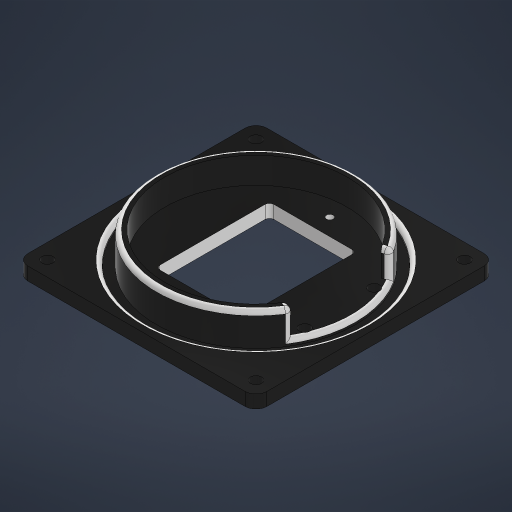
# Autodesk Inventor part: UnitV_Mount
Saved by Autodesk Inventor 2024.2 (Build 282272000, 272)
## iProperties
Created: 2024-02-19
Part Number: UnitV_Mount
Material: 一般
Document SubType Name: Modeling
Designer: Hanaoka
Density: 1 g/cm^3
Appearance: 既定
Author: Hanaoka
Autodesk Inventor part; units mm, degrees
ref_plane "YZ Plane" through (0, 0, 0) normal (1, 0, 0) x (0, 1, 0)
ref_plane "XZ Plane" through (0, 0, 0) normal (0, 1, 0) x (-1, 0, 0)
ref_plane "XY Plane" through (0, 0, 0) normal (0, 0, 1) x (1, 0, 0)
sketch "スケッチ1" plane through (0, 0, 0) normal (0, 1, 0) x (-1, 0, 0)
  line L0 (-24, 24) -> (24, 24) construction
  line L1 (24, 24) -> (24, -24) construction
  line L2 (24, -24) -> (-24, -24) construction
  line L3 (-24, -24) -> (-24, 24) construction
  line L4 (-24, 24) -> (24, -24) construction
  line L5 (24, 24) -> (-24, -24) construction
  line L6 (-25, 27.5) -> (25, 27.5)
  line L7 (27.5, 25) -> (27.5, -25)
  line L8 (25, -27.5) -> (-25, -27.5)
  line L9 (-27.5, -25) -> (-27.5, 25)
  line L10 (-27.5, 27.5) -> (27.5, -27.5) construction
  line L11 (27.5, 27.5) -> (-27.5, -27.5) construction
  arc A0 (27.5, 25) -> (25, 27.5) centre (25, 25) ccw
  arc A1 (25, -27.5) -> (27.5, -25) centre (25, -25) ccw
  arc A2 (-27.5, -25) -> (-25, -27.5) centre (-25, -25) ccw
  arc A3 (-25, 27.5) -> (-27.5, 25) centre (-25, 25) ccw
  circle A4 centre (24, 24) radius 1.3
  circle A5 centre (24, -24) radius 1.3
  circle A6 centre (-24, 24) radius 1.3
  circle A7 centre (-24, -24) radius 1.3
  point P0 (0, 0)
  dimension "d0" = 48
  dimension "d1" = 48
  dimension "d2" = 2.5
  dimension "d3" = 2.6
  dimension "d55" = 55
  constraints: 24 end point, 12 point on line, 8 centre point, 8 point on circle, 8 tangent, 6 equal radius, 4 midpoint, 4 parallel, 2 horizontal, 2 perpendicular, 1 coincident
  measures "d0" distance of L0.start L0.end
  measures "d1" distance of L1.end L0.end
  measures "d2" radius of A0
  measures "d3" diameter of A6
  measures "d55" distance between parallel lines of L7 L9
extrude "押し出し1" add sketch "スケッチ1" along normal blind 3
sketch "スケッチ2" plane through (0, 3, 0) normal (0, 1, 0) x (1, 0, 0)
  circle A0 centre (0, 0) radius 22.9
  line L0 (25, 27.5) -> (-25, 27.5) projected
  arc A1 (-25, 27.5) -> (-27.5, 25) centre (-25, 25) ccw projected
  line L1 (-27.5, 25) -> (-27.5, -25) projected
  arc A2 (-27.5, -25) -> (-25, -27.5) centre (-25, -25) ccw projected
  line L2 (-25, -27.5) -> (25, -27.5) projected
  arc A3 (25, -27.5) -> (27.5, -25) centre (25, -25) ccw projected
  line L3 (27.5, -25) -> (27.5, 25) projected
  arc A4 (27.5, 25) -> (25, 27.5) centre (25, 25) ccw projected
  circle A5 centre (24, 24) radius 1.3 projected
  circle A6 centre (24, -24) radius 1.3 projected
  circle A7 centre (-24, 24) radius 1.3 projected
  circle A8 centre (-24, -24) radius 1.3 projected
  circle A9 centre (0, 0) radius 25.05
  circle A10 centre (0, 0) radius 21
  dimension "d7" = 45.8
  dimension "d9" = 50.1
  dimension "d10" = 42
  constraints: 3 centre point, 2 coincident
  measures "d7" diameter of A0
  measures "d9" diameter of A9
  measures "d10" diameter of A10
extrude "押し出し2" cut sketch "スケッチ2" against normal blind 1.5 contours A9
extrude "押し出し6" add sketch "スケッチ2" along normal blind 6 contours A0
sketch "スケッチ5" plane through (0, 3, 0) normal (0, 1, 0) x (1, 0, 0)
  line L0 (9, -12.1) -> (-9, -12.1)
  line L1 (-9, -12.1) -> (-9, 12.1)
  line L2 (-9, 12.1) -> (9, 12.1)
  line L3 (9, 12.1) -> (9, -12.1)
  line L4 (9, -12.1) -> (-9, 12.1) construction
  line L5 (-9, -12.1) -> (9, 12.1) construction
  circle A0 centre (19.2, -8) radius 1.25
  circle A1 centre (19.2, 8) radius 1.25
  line L6 (31, 12) -> (-9, 12) construction
  line L7 (-9, -12) -> (31, -12) construction
  line L8 (31, -12) -> (31, 12) construction
  line L9 (31, 12) -> (-9, -12) construction
  line L10 (-9, 12) -> (31, -12) construction
  line L11 (0, 0) -> (27.5, 0) construction
  line L12 (27.5, -25) -> (27.5, 25) projected
  line L13 (19.2, -8) -> (19.2, 8) construction
  circle A2 centre (19.2, -8) radius 3
  circle A3 centre (19.2, 8) radius 3
  circle A4 centre (0, 0) radius 22.9 projected
  circle A5 centre (0, 0) radius 21 projected
  point P0 (11, 0)
  point P1 (20.3396, -5.2249)
  point P2 (21.9002, -6.6927)
  point P3 (21.9002, 6.6927)
  point P4 (20.3396, 5.2249)
  dimension "d33" = 18
  dimension "d34" = 24.2
  dimension "d35" = 2.5
  dimension "d37" = 24
  dimension "d38" = 40
  dimension "d39" = 11.8
  dimension "d40" = 16
  dimension "d41" = 6
  constraints: 26 end point, 5 midpoint, 4 centre point, 3 parallel, 2 coincident, 2 equal radius, 2 horizontal, 1 perpendicular, 1 point on line, 1 vertical, 2 other
  measures "d33" distance of L1.end L2.end
  measures "d34" distance of L0.end L1.end
  measures "d35" diameter of A0
  measures "d37" distance of L7.end L6.start
  measures "d38" distance of L6.start L6.end
  measures "d39" distance between parallel lines of L8 L13
  measures "d40" distance of L13.start L13.end
  measures "d41" diameter of A2
extrude "押し出し7" cut sketch "スケッチ5" along normal up to surface (6 mm away) contours A0 A5 | A0 A5 A2 A4 | A5 A0 | A0 A5 A2 | A5 A3 A4 A2 | A2 A4 | A5 A1 A3 | A3 A4 A5 A1 | A3 A4 | A5 A1 | A1 A5 picked at (22.2048, -1.3394)
extrude "押し出し8" cut sketch "スケッチ5" against normal up to surface (3 mm away) contours L0 L1 L2 L3 | A0 A5 | A5 A0 | A5 A1 | A1 A5
sketch "スケッチ6" plane through (0, 3, 0) normal (0, 1, 0) x (1, 0, 0)
  circle A0 centre (19.2, 8) radius 1.25 projected
  line L0 (-9, 12.1) -> (9, 12.1) projected
  line L1 (9, 12.1) -> (9, -12.1) projected
  line L2 (9, -12.1) -> (-9, -12.1) projected
  line L3 (-9, -12.1) -> (-9, 12.1) projected
  circle A1 centre (19.2, -8) radius 1.25 projected
  arc A2 (18.032, -10.7633) -> (20.173, -10.8378) centre (19.2, -8) ccw projected
  arc A3 (20.173, -10.8378) -> (20.173, 10.8378) centre (0, 0) ccw projected
  arc A4 (20.173, 10.8378) -> (18.032, 10.7633) centre (19.2, 8) ccw projected
  arc A5 (18.032, 10.7633) -> (18.032, -10.7633) centre (0, 0) ccw projected
  line L4 (10, -13.1) -> (-10, -13.1)
  line L5 (-10, -13.1) -> (-10, 13.1)
  line L6 (-10, 13.1) -> (10, 13.1)
  line L7 (10, 13.1) -> (10, -13.1)
  line L8 (10, -13.1) -> (-10, 13.1) construction
  line L9 (-10, -13.1) -> (10, 13.1) construction
  dimension "d46" = 1
  dimension "d47" = 1
  constraints: 12 end point, 2 midpoint, 2 parallel, 1 horizontal, 1 perpendicular
  measures "d46" distance between parallel lines of L4 L2
  measures "d47" distance between parallel lines of L3 L5
extrude "押し出し9" cut sketch "スケッチ6" against normal up to surface (3 mm away) contours L4 L5 L6 L7
fillet "フィレット1" radius 1 6 edges at (-10, 1.5, 13.1) (10, 1.5, 13.1) (10, 1.5, -13.1) (-10, 1.5, -13.1) (20.173, 6, 10.8378) (20.173, 6, -10.8378)
sketch "スケッチ7" plane through (0, 0, 0) normal (0, -1, 0) x (1, 0, 0)
  line L0 (9, -13.1) -> (-9, -13.1) projected
  arc A0 (-10, -12.1) -> (-9, -13.1) centre (-9, -12.1) ccw projected
  line L1 (-10, -12.1) -> (-10, 12.1) projected
  arc A1 (-9, 13.1) -> (-10, 12.1) centre (-9, 12.1) ccw projected
  line L2 (-9, 13.1) -> (9, 13.1) projected
  arc A2 (10, 12.1) -> (9, 13.1) centre (9, 12.1) ccw projected
  line L3 (10, 12.1) -> (10, -12.1) projected
  arc A3 (9, -13.1) -> (10, -12.1) centre (9, -12.1) ccw projected
  circle A4 centre (19.2, -8) radius 1.25 projected
  circle A5 centre (19.2, 8) radius 1.25 projected
  line L4 (25, -27.5) -> (-25, -27.5) projected
  arc A6 (25, -27.5) -> (27.5, -25) centre (25, -25) ccw projected
  line L5 (27.5, 25) -> (27.5, -25) projected
  arc A7 (27.5, 25) -> (25, 27.5) centre (25, 25) ccw projected
  line L6 (-25, 27.5) -> (25, 27.5) projected
  arc A8 (-25, 27.5) -> (-27.5, 25) centre (-25, 25) ccw projected
  line L7 (-27.5, -25) -> (-27.5, 25) projected
  arc A9 (-27.5, -25) -> (-25, -27.5) centre (-25, -25) ccw projected
  circle A10 centre (24, -24) radius 1.3 projected
  circle A11 centre (24, 24) radius 1.3 projected
  circle A12 centre (-24, -24) radius 1.3 projected
  circle A13 centre (-24, 24) radius 1.3 projected
  line L8 (9, -13.1) -> (23, -13.1)
  line L9 (23, -13.1) -> (23, 13.1)
  line L10 (23, 13.1) -> (9, 13.1)
  line L11 (10, 12.1) -> (10, -12.1) projected
  point P0 (0, 0)
  dimension "d52" = 14
  constraints: 6 end point, 2 parallel, 1 horizontal
  measures "d52" distance of L0.start L8.end
extrude "押し出し10" add sketch "スケッチ7" along normal blind 1.5 contours A3 L3 A2 L10 L9 L8
fillet "フィレット2" radius 1 8 edges at (-25.05, 3, 0) (19.299, 9, 11.5302) (18.3027, 9, 10.8627) (19.299, 9, -11.5302) (18.3027, 9, -10.8627) (-22.9, 9, 0) (23, -0.75, -13.1) (23, -0.75, 13.1)
sketch "スケッチ8" plane through (0, 3, 0) normal (0, 1, 0) x (1, 0, 0)
  circle A0 centre (0, -17) radius 0.8
  line L0 (-38.5, 0) -> (38.5, 0) construction
  line L1 (0, 38.5) -> (0, -38.5) construction
  circle A1 centre (0, 17) radius 0.8
  point P0 (0, 0)
  dimension "d57" = 1.6
  dimension "d58" = 34
  constraints: 2 centre point, 1 point on line, 1 symmetric about line, 1 other
  measures "d57" diameter of A0
  measures "d58" distance of A1.centre A0.centre
extrude "押し出し11" cut sketch "スケッチ8" against normal up to surface (3 mm away)
fillet "フィレット3" radius 1 2 edges at (21.9594, 3, -6.4959) (21.9594, 3, 6.4959)
equation "\"d47\" = d46"
